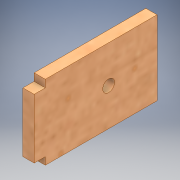
# Autodesk Inventor part: Podstawa - drugie mocowanie
Saved by Autodesk Inventor 2017 (Build 210142000, 142)
## iProperties
Created: 2017-05-18
Part Number: Podstawa - drugie mocowanie
Material: Drewno (wiśnia)
Document SubType Name: Modeling
Designer: Damian
Density: 0.63 g/cm^3
Appearance: Wiśnia — naturalna — niski połysk
Author: Damian
Autodesk Inventor part; units mm, degrees
ref_plane "YZ Plane" through (0, 0, 0) normal (1, 0, 0) x (0, 1, 0)
ref_plane "XZ Plane" through (0, 0, 0) normal (0, 1, 0) x (-1, 0, 0)
ref_plane "XY Plane" through (0, 0, 0) normal (0, 0, 1) x (1, 0, 0)
sketch "Szkic1" plane through (0, 0, 0) normal (1, 0, 0) x (0, 1, 0)
  line L0 (0, 0) -> (30, 0)
  line L1 (30, 0) -> (30, 20)
  line L2 (30, 20) -> (0, 20)
  circle A0 centre (17, 10) radius 1.6
  line L3 (0, 18) -> (-3, 18)
  line L4 (-3, 18) -> (-3, 2)
  line L5 (-3, 2) -> (0, 2)
  line L6 (0, 20) -> (0, 18)
  line L7 (0, 2) -> (0, 0)
  dimension "d0" = 30
  dimension "d1" = 20
  dimension "d2" = 13
  dimension "d3" = 3.2
  dimension "d6" = 2
  constraints: 16 end point, 4 parallel, 2 horizontal, 2 perpendicular, 1 centre point, 1 coincident
  measures "d0" distance of L2.end L1.end
  measures "d1" distance of L1.end L0.end
  measures "d2" distance from line of L1 point (17, 10)
  measures "d3" diameter of A0
  measures "d6" distance between parallel lines of L2 L3
extrude "Wyciągnięcie proste1" add sketch "Szkic1" along normal blind 3
